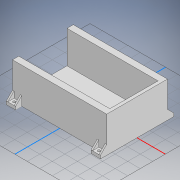
# Autodesk Inventor part: 000.003.001 - Основание
Saved by Autodesk Inventor 2022 (Build 260153000, 153)
## iProperties
Created: 2022-02-26
Part Number: 000.003.001 - Основание
Material: Типовые
Document SubType Name: Modeling
Designer: Petrov Ivan
Density: 1 g/cm^3
Appearance: По умолчанию
Author: Petrov Ivan
Autodesk Inventor part; units mm, degrees
ref_plane "YZ Plane" through (0, 0, 0) normal (1, 0, 0) x (0, 1, 0)
ref_plane "XZ Plane" through (0, 0, 0) normal (0, 1, 0) x (-1, 0, 0)
ref_plane "XY Plane" through (0, 0, 0) normal (0, 0, 1) x (1, 0, 0)
sketch "Эскиз1" plane through (0, 0, 0) normal (0, 1, 0) x (-1, 0, 0)
  line L0 (75, 48.402) -> (-75, 48.402)
  line L1 (-75, 48.402) -> (-75, -48.402)
  line L2 (-75, -48.402) -> (75, -48.402)
  line L3 (75, -48.402) -> (75, 48.402)
  point P0 (0, 0)
  dimension "d0" = 150
  dimension "d1" = 96.804
  dimension "d29" = 48.402
  dimension "d30" = 75
  constraints: 8 end point, 2 parallel, 1 horizontal, 1 perpendicular
  measures "d0" distance of L2.end L1.end
  measures "d1" distance of L1.end L0.end
  measures "d29" distance from line of point (0, 0) L2
  measures "d30" distance from line of point (0, 0) L1
extrude "Выдавливание1" add sketch "Эскиз1" along normal blind 5
sketch "Эскиз3" plane through (0, 5, 0) normal (0, 1, 0) x (1, 0, 0)
  line L0 (-75, 48.402) -> (-75, -48.402) projected
  line L1 (-75, 48.402) -> (-75, 38.402)
  line L2 (-75, 38.402) -> (70, 38.402)
  line L3 (70, 38.402) -> (70, -38.402)
  line L4 (70, -38.402) -> (-75, -38.402)
  line L5 (-75, -48.402) -> (75, -48.402) projected
  line L6 (75, 48.402) -> (-75, 48.402) projected
  line L7 (75, -48.402) -> (75, 48.402) projected
  point P0 (0, 0)
  point P1 (-75, -38.402)
  dimension "d11" = 10
  dimension "d12" = 10
  dimension "d13" = 5
  constraints: 8 end point, 2 perpendicular, 2 point on line, 1 horizontal
  measures "d11" distance between parallel lines of L4 L5
  measures "d12" distance between parallel lines of L6 L2
  measures "d13" distance between parallel lines of L7 L3
extrude "Выдавливание3" add sketch "Эскиз3" along normal blind 51.75 contours L6 L7 L5 L0 L4 L3 L2
sketch "Эскиз4" plane through (0, 0, 0) normal (0, -1, 0) x (1, 0, 0)
  line L0 (-75, 48.402) -> (75, 48.402) projected
  line L1 (75, 48.402) -> (60, 48.402)
  line L2 (60, 48.402) -> (60, 58.402)
  line L3 (60, 58.402) -> (75, 58.402)
  line L4 (75, 58.402) -> (75, 48.402)
  circle A0 centre (67.5, 53.402) radius 2
  point P0 (0, 0)
  point P1 (67.5, 58.402)
  dimension "d16" = 15
  dimension "d17" = 10
  dimension "d18" = 4
  constraints: 8 end point, 2 parallel, 1 centre point, 1 horizontal, 1 midpoint, 1 perpendicular, 1 vertical alignment
  measures "d16" distance of L2.end L3.end
  measures "d17" distance of L1.end L2.end
  measures "d18" diameter of A0
extrude "Выдавливание4" add sketch "Эскиз4" against normal blind 5
sketch "Эскиз5" plane through (0, 5, 0) normal (0, 1, 0) x (1, 0, 0)
  line L0 (60, -48.402) -> (60, -58.402) projected
  line L1 (-75, -48.402) -> (75, -48.402) projected
  line L2 (60, -58.402) -> (62.5, -58.402)
  line L3 (62.5, -58.402) -> (62.5, -48.402)
  line L4 (62.5, -48.402) -> (60, -48.402)
  line L5 (60, -48.402) -> (60, -58.402)
  line L6 (75, -58.402) -> (75, 48.402) projected
  line L7 (75, -58.402) -> (72.5, -58.402)
  line L8 (72.5, -58.402) -> (72.5, -48.402)
  line L9 (72.5, -48.402) -> (75, -48.402)
  line L10 (75, -48.402) -> (75, -58.402)
  point P0 (0, 0)
  dimension "d21" = 2.5
  dimension "d22" = 2.5
  constraints: 16 end point, 4 parallel, 2 horizontal, 2 perpendicular, 2 point on line
  measures "d21" distance between parallel lines of L0 L3
  measures "d22" distance between parallel lines of L6 L8
extrude "Выдавливание5" add sketch "Эскиз5" along normal blind 10
chamfer "Фаска1" distance 10 angle 45 2 edges at (61.25, 15, 58.402) (73.75, 15, 58.402)
mirror "Зеркальное отражение1" about plane through (0, 0, 0) normal (1, 0, 0) of "Выдавливание5", "Выдавливание4", "Фаска1"
mirror "Зеркальное отражение2" about plane through (0, 0, 0) normal (0, 0, 1) of "Выдавливание5", "Выдавливание4", "Фаска1", "Зеркальное отражение1"
equation "\"d29\" = 0.5 * d1"
equation "\"d30\" = 0.5 * d0"
equation "\"d12\" = d11"
